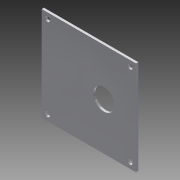
# Autodesk Inventor part: gearboxbearingplate(gbpb)
Saved by Autodesk Inventor 2015 (Build 190159000, 159)
## iProperties
Created: 2015-10-03
Part Number: gearboxbearingplate(gbpb)
Material: Aluminum 6061
Document SubType Name: Sheet Metal
Designer: elilitwack
Density: 2.7 g/cm^3
Sheet Metal Rule: Default
Appearance: Aluminum - Flat
Mass: 126.415 g
Surface Area: 327.873 cm^2
Volume: 46.8204 cm^3
RuleStatus: InUse
Author: elilitwack
Autodesk Inventor part; units mm, degrees
ref_plane "YZ Plane" through (0, 0, 0) normal (1, 0, 0) x (0, 1, 0)
ref_plane "XZ Plane" through (0, 0, 0) normal (0, 1, 0) x (-1, 0, 0)
ref_plane "XY Plane" through (0, 0, 0) normal (0, 0, 1) x (1, 0, 0)
sketch "Sketch1" plane through (0, 0, 0) normal (0, 0, 1) x (1, 0, 0)
  line L0 (0, 0) -> (127, 0)
  line L1 (127, 0) -> (127, 127)
  line L2 (127, 127) -> (0, 127)
  line L3 (0, 127) -> (0, 0)
  dimension "d0" = 127
  constraints: 8 end point, 2 parallel, 2 perpendicular, 1 horizontal
  measures "d0" distance of L2.end L0.start
extrude "Plate1" add sketch "Sketch1" along normal blind 3.048
sketch "gbmh_sketch" plane through (0, 0, 3.048) normal (0, 0, 1) x (1, 0, 0)
  line L0 (7.9375, 119.0625) -> (119.0625, 119.0625) construction
  line L1 (127, 127) -> (0, 127) construction
  line L2 (119.0625, 119.0625) -> (119.0625, 7.9375) construction
  line L3 (119.0625, 7.9375) -> (7.9375, 7.9375) construction
  line L4 (7.9375, 7.9375) -> (7.9375, 119.0625) construction
  line L5 (7.9375, 119.0625) -> (7.9375, 127) construction
  line L6 (7.9375, 119.0625) -> (0, 119.0625) construction
  line L7 (0, 127) -> (0, 0) construction
  line L8 (119.0625, 7.9375) -> (127, 7.9375) construction
  line L9 (127, 0) -> (127, 127) construction
  line L10 (119.0625, 7.9375) -> (119.0625, 0) construction
  dimension "d2" = 111.1504
  dimension "d3" = 111.1504
  dimension "d4" = 111.1504
  dimension "d5" = 111.1504
  constraints: 16 end point, 5 perpendicular, 4 point on line, 1 horizontal, 1 parallel, 1 vertical
hole "gbmh" at (7.9375, 119.0625, 3.048) at (7.9375, 7.9375, 3.048) at (119.0625, 7.9375, 3.048) at (119.0625, 119.0625, 3.048) direction (0, 0, -1) diameter 6.35 depth 3.048 tip angle 118
sketch "bearing_hole_sketch" plane through (0, 0, 3.048) normal (0, 0, 1) x (1, 0, 0)
  line L0 (127, 0) -> (0, 0) projected
  line L1 (127, 127) -> (127, 0) projected
  point P0 (83.8454, 63.5)
  dimension "d13" = 38.1
  dimension "d14" = 38.1
hole "ss_bearing_hole" at (83.8454, 63.5, 3.048) direction (0, 0, -1) diameter 28.575 depth 3.048 tip angle 118
equation "\"d6\" = gb_mh_diameter"
equation "\"d11\" = Thickness"
equation "\"d15\" = gb_bearing_diameter"
equation "\"d20\" = Thickness"
equation "\"BendRadius\" = Thickness"
equation "\"BendReliefWidth\" = Thickness"
equation "\"BendReliefDepth\" = 0.5 * Thickness"
equation "\"CornerReliefSize\" = 4 * Thickness"
equation "\"MinimumRemnant\" = 2 * Thickness"
equation "\"TransitionRadius\" = BendRadius"
equation "\"JacobiRadiusSize\" = BendRadius"
equation "\"GapSize\" = Thickness"
equation "\"d1\" = BendRadius"
equation "\"gb_mh_seperation\" = 111.1504"
equation "\"gb_mh_diameter\" = 6.35"
equation "\"gb_axle_from_edge\" = 38.1"
equation "\"gb_width\" = 127"
equation "\"gb_bearing_diameter\" = 28.575"
equation "\"gb_to_bottom_of_side_assembly\" = 4.7752"
equation "\"gb_mh_seperation_alt\" = 111.125"
equation "\"gb_axle_from_edge_alt\" = 43.1546"
equation "\"Thickness\" = 3.048"
body "Solid1"
